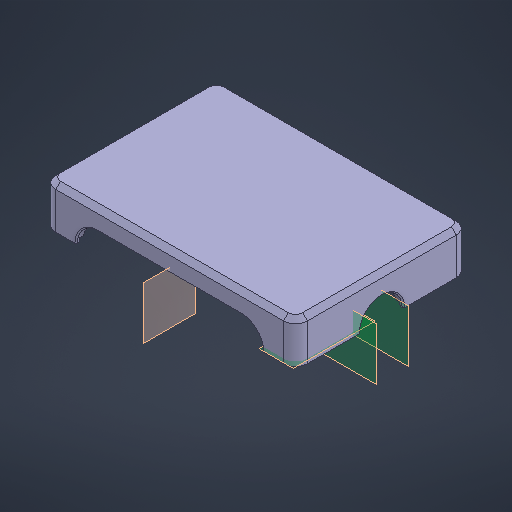
# Autodesk Inventor part: case2
Saved by Autodesk Inventor 2025.2 (Build 292293000, 293)
## iProperties
Created: 2025-10-05
Part Number: case2
Material: Generic
Document SubType Name: Modeling
Designer: micyg
Density: 1 g/cm^3
Appearance: Default
Sheet Metal Rule: Default
Author: micyg
## iProperties of the stored document case2_3DPrint.ipt
Created: 2025-10-05
Part Number: case2_3DPrint
Material: Generic
Document SubType Name: Modeling
Designer: micyg
Density: 1 g/cm^3
Appearance: Default
Author: micyg
Autodesk Inventor part; units mm, degrees
ref_plane "YZ Plane" through (0, 0, 0) normal (1, 0, 0) x (0, 1, 0)
ref_plane "XZ Plane" through (0, 0, 0) normal (0, 1, 0) x (-1, 0, 0)
ref_plane "XY Plane" through (0, 0, 0) normal (0, 0, 1) x (1, 0, 0)
sketch "Sketch1" plane through (0, 0, 0) normal (0, 1, 0) x (-1, 0, 0)
  line L0 (0, 0) -> (105.2, 0)
  line L1 (105.2, 0) -> (105.2, -72.2)
  line L2 (105.2, -72.2) -> (0, -72.2)
  line L3 (0, -72.2) -> (0, 0)
  dimension "d0" = 105.2
  dimension "d1" = 72.2
  constraints: 8 end point, 2 parallel, 1 horizontal, 1 perpendicular
  measures "d0" distance of L1.end L2.end
  measures "d1" distance of L0.end L1.end
extrude "Extrusion1" add sketch "Sketch1" along normal blind 17.5
fillet "Fillet1" radius 5 4 edges at (-105.2, 8.75, 0) (0, 8.75, 0) (-105.2, 8.75, -72.2) (0, 8.75, -72.2)
chamfer "Chamfer1" distance 2 angle 45 8 edges at (-52.6, 17.5, 0) (-1.4645, 17.5, -1.4645) (0, 17.5, -36.1) (-1.4645, 17.5, -70.7355) (-52.6, 17.5, -72.2) (-103.7355, 17.5, -70.7355) (-105.2, 17.5, -36.1) (-103.7355, 17.5, -1.4645)
shell "Shell2" thickness 3 removed faces 1 at (-36.7333, 0, -24.0667)
ref_plane "Work Plane2" through (-52.6, 0, 0) normal (1, 0, 0) x (0, 1, 0)
ref_plane "Work Plane3" through (0, 0, -36.1) normal (0, 0, -1) x (-1, 0, 0)
ref_plane "Work Plane4" through (0, 1.915, 0) normal (0, -1, 0) x (1, 0, 0)
sketch "Sketch19" plane through (-52.6, 0, 0) normal (1, 0, 0) x (0, 1, 0)
  line L0 (0, -3) -> (14.2574, -3) projected
  line L1 (14.2574, -3) -> (0, -3) projected
  line L2 (14.5, -5.7) -> (7.5, -5.7)
  line L3 (6.5, -5.7) -> (7.5, -6.7) construction
  line L4 (7.5, -6.7) -> (7.5, -5.7)
  line L5 (7.5, -5.7) -> (6.5, -5.7) construction
  line L6 (7.5, -6.7) -> (14.5, -13.7)
  line L7 (0, -67.2) -> (0, -72.2) projected
  line L8 (0, -5) -> (0, -67.2) projected
  line L9 (0, 0) -> (0, -5) projected
  line L10 (0, -5) -> (0, 0) projected
  line L11 (0, -67.2) -> (0, -5) projected
  line L12 (0, -72.2) -> (0, -67.2) projected
  line L13 (14.5, -3.2426) -> (14.5, -5) projected
  line L14 (14.5, -5) -> (14.5, -67.2) projected
  line L15 (14.5, -67.2) -> (14.5, -68.9574) projected
  line L16 (14.5, -68.9574) -> (14.5, -67.2) projected
  line L17 (14.5, -67.2) -> (14.5, -5) projected
  line L18 (14.5, -5) -> (14.5, -3.2426) projected
  dimension "d104" = 2.7
  dimension "d105" = 1
  dimension "d157" = 45
  dimension "d179" = 7
  constraints: 10 end point, 2 perpendicular, 2 point on line, 1 collinear
  measures "d104" distance between parallel lines of L0 L2
  measures "d105" distance from line of L3.end L2
  measures "d157" angle of L17 L6
  measures "d179" distance between parallel lines of L17 L4
extrude "Extrusion15" add sketch "Sketch19" against normal up to surface (49.6 mm away)
mirror "Mirror9" about plane through (-52.6, 0, 0) normal (1, 0, 0) of "Extrusion15"
mirror "Mirror10" about plane through (0, 0, -36.1) normal (0, 0, -1) of "Extrusion15", "Mirror9"
sketch "Sketch9" plane through (0, 1.915, 0) normal (0, -1, 0) x (1, 0, 0)
  arc A0 (-5, -72.2) -> (0, -67.2) centre (-5, -67.2) ccw projected
  line L0 (0, -5) -> (0, -67.2) projected
  arc A1 (0, -5) -> (-5, 0) centre (-5, -5) ccw projected
  line L1 (-100.2, 0) -> (-5, 0) projected
  arc A2 (-100.2, 0) -> (-105.2, -5) centre (-100.2, -5) ccw projected
  line L2 (-105.2, -67.2) -> (-105.2, -5) projected
  arc A3 (-105.2, -67.2) -> (-100.2, -72.2) centre (-100.2, -67.2) ccw projected
  line L3 (-5, -72.2) -> (-100.2, -72.2) projected
  line L4 (-5, -70.8) -> (-100.2, -70.8) projected
  arc A4 (-5, -70.8) -> (-1.4, -67.2) centre (-5, -67.2) ccw projected
  line L5 (-1.4, -5) -> (-1.4, -67.2) projected
  arc A5 (-1.4, -5) -> (-5, -1.4) centre (-5, -5) ccw projected
  line L6 (-100.2, -1.4) -> (-5, -1.4) projected
  arc A6 (-100.2, -1.4) -> (-103.8, -5) centre (-100.2, -5) ccw projected
  line L7 (-103.8, -67.2) -> (-103.8, -5) projected
  arc A7 (-103.8, -67.2) -> (-100.2, -70.8) centre (-100.2, -67.2) ccw projected
  line L8 (-102.2, -5) -> (-102.2, -67.2) projected
  arc A8 (-100.2, -3) -> (-102.2, -5) centre (-100.2, -5) ccw projected
  line L9 (-5, -3) -> (-100.2, -3) projected
  arc A9 (-3, -5) -> (-5, -3) centre (-5, -5) ccw projected
  line L10 (-3, -67.2) -> (-3, -5) projected
  arc A10 (-5, -69.2) -> (-3, -67.2) centre (-5, -67.2) ccw projected
  line L11 (-100.2, -69.2) -> (-5, -69.2) projected
  arc A11 (-102.2, -67.2) -> (-100.2, -69.2) centre (-100.2, -67.2) ccw projected
  line L12 (-96.7, -8.6) -> (-8.7, -8.6) construction
  line L13 (-8.7, -8.6) -> (-8.7, -63.6) construction
  line L14 (-8.7, -63.6) -> (-96.7, -63.6) construction
  line L15 (-96.7, -63.6) -> (-96.7, -8.6) construction
  circle A12 centre (-96.7, -8.6) radius 1.5
  circle A13 centre (-8.7, -8.6) radius 1.5
  circle A14 centre (-96.7, -63.6) radius 1.5
  circle A15 centre (-8.7, -63.6) radius 1.5
  line L16 (-52.7, -8.6) -> (-52.7, -63.6) construction
  line L17 (-101.7, -3.6) -> (-3.7, -3.6) construction
  line L18 (-3.7, -3.6) -> (-3.7, -68.6) construction
  line L19 (-3.7, -68.6) -> (-101.7, -68.6) construction
  line L20 (-101.7, -68.6) -> (-101.7, -3.6) construction
  line L21 (-101.7, -36.1) -> (-3.7, -36.1) construction
  line L22 (-52.6, 0) -> (-52.6, -72.2) construction
  line L23 (-105.2, -36.1) -> (0, -36.1) construction
  line L24 (-93.2, -3) -> (-93.2, -8.6)
  line L25 (-102.2, -12.1) -> (-102.2, -5)
  arc A16 (-96.7, -12.1) -> (-93.2, -8.6) centre (-96.7, -8.6) ccw
  line L26 (-96.7, -12.1) -> (-102.2, -12.1)
  line L27 (-100.2, -3) -> (-93.2, -3)
  line L28 (-93.2, -69.2) -> (-93.2, -63.6)
  arc A17 (-93.2, -63.6) -> (-96.7, -60.1) centre (-96.7, -63.6) ccw
  line L29 (-96.7, -60.1) -> (-102.2, -60.1)
  arc A18 (-12.2, -8.6) -> (-8.7, -12.1) centre (-8.7, -8.6) ccw
  line L30 (-3, -12.1) -> (-3, -5)
  line L31 (-12.2, -3) -> (-12.2, -8.6)
  line L32 (-8.7, -12.1) -> (-3, -12.1)
  line L33 (-5, -3) -> (-12.2, -3)
  arc A19 (-8.7, -60.1) -> (-12.2, -63.6) centre (-8.7, -63.6) ccw
  line L34 (-12.2, -69.2) -> (-12.2, -63.6)
  line L35 (-8.7, -60.1) -> (-3, -60.1)
  line L36 (-93.2, -3) -> (-95.2, -3)
  line L37 (-95.2, -3) -> (-95.2, -6)
  line L38 (-95.2, -6) -> (-93.2, -6)
  line L39 (-93.2, -6) -> (-93.2, -3)
  line L40 (-12.2, -3) -> (-10.2, -3)
  line L41 (-10.2, -3) -> (-10.2, -6)
  line L42 (-10.2, -6) -> (-12.2, -6)
  line L43 (-12.2, -6) -> (-12.2, -3)
  line L44 (-95.2, -69.2) -> (-95.2, -66.2)
  line L45 (-95.2, -66.2) -> (-93.2, -66.2)
  line L46 (-10.2, -69.2) -> (-10.2, -66.2)
  line L47 (-10.2, -66.2) -> (-12.2, -66.2)
  arc A20 (-3, -5) -> (-5, -3) centre (-5, -5) ccw projected
  line L48 (-5, -3) -> (-100.2, -3) projected
  arc A21 (-100.2, -3) -> (-102.2, -5) centre (-100.2, -5) ccw projected
  line L49 (-102.2, -5) -> (-102.2, -67.2) projected
  arc A22 (-102.2, -67.2) -> (-100.2, -69.2) centre (-100.2, -67.2) ccw projected
  line L50 (-100.2, -69.2) -> (-5, -69.2) projected
  arc A23 (-5, -69.2) -> (-3, -67.2) centre (-5, -67.2) ccw projected
  line L51 (-3, -67.2) -> (-3, -5) projected
  arc A24 (0, -5) -> (-5, 0) centre (-5, -5) ccw projected
  line L52 (0, -5) -> (0, -67.2) projected
  arc A25 (-5, -72.2) -> (0, -67.2) centre (-5, -67.2) ccw projected
  line L53 (-5, -72.2) -> (-100.2, -72.2) projected
  arc A26 (-105.2, -67.2) -> (-100.2, -72.2) centre (-100.2, -67.2) ccw projected
  line L54 (-105.2, -67.2) -> (-105.2, -5) projected
  arc A27 (-100.2, 0) -> (-105.2, -5) centre (-100.2, -5) ccw projected
  line L55 (-100.2, 0) -> (-5, 0) projected
  arc A28 (-3, -5) -> (-5, -3) centre (-5, -5) ccw projected
  line L56 (-5, -3) -> (-100.2, -3) projected
  arc A29 (-100.2, -3) -> (-102.2, -5) centre (-100.2, -5) ccw projected
  line L57 (-102.2, -5) -> (-102.2, -67.2) projected
  arc A30 (-102.2, -67.2) -> (-100.2, -69.2) centre (-100.2, -67.2) ccw projected
  line L58 (-100.2, -69.2) -> (-5, -69.2) projected
  arc A31 (-5, -69.2) -> (-3, -67.2) centre (-5, -67.2) ccw projected
  line L59 (-3, -67.2) -> (-3, -5) projected
  arc A32 (0, -5) -> (-5, 0) centre (-5, -5) ccw projected
  line L60 (0, -5) -> (0, -67.2) projected
  arc A33 (-5, -72.2) -> (0, -67.2) centre (-5, -67.2) ccw projected
  line L61 (-5, -72.2) -> (-100.2, -72.2) projected
  arc A34 (-105.2, -67.2) -> (-100.2, -72.2) centre (-100.2, -67.2) ccw projected
  line L62 (-105.2, -67.2) -> (-105.2, -5) projected
  arc A35 (-100.2, 0) -> (-105.2, -5) centre (-100.2, -5) ccw projected
  line L63 (-100.2, 0) -> (-5, 0) projected
  point P0 (-52.7, -36.1)
  dimension "d137" = 88
  dimension "d138" = 55
  dimension "d139" = 3
  dimension "d140" = 3
  dimension "d141" = 3
  dimension "d142" = 3
  dimension "d143" = 98
  dimension "d144" = 65
  dimension "d145" = 0.5
  dimension "d147" = 2
  dimension "d148" = 2
  dimension "d149" = 3
  dimension "d150" = 2
  constraints: 72 end point, 16 symmetric about line, 12 parallel, 12 point on circle, 10 midpoint, 8 centre point, 6 horizontal, 6 perpendicular, 6 point on line, 5 coincident, 4 tangent, 1 collinear, 3 other
  measures "d137" distance of L12.start L12.end
  measures "d138" distance of L14.end L12.start
  measures "d139" diameter of A12
  measures "d140" diameter of A15
  measures "d141" diameter of A13
  measures "d142" diameter of A14
  measures "d143" distance of L17.start L17.end
  measures "d144" distance of L19.end L17.start
  measures "d145" distance between parallel lines of L8 L20
  measures "d147" radial gap between concentric circles of A12 A16
  measures "d148" radial gap between concentric circles of A18 A13
  measures "d149" distance between parallel lines of L9 L38
  measures "d150" distance between parallel lines of L24 L37
extrude "Extrusion13" add sketch "Sketch9" against normal up to surface (12.585 mm away) contours A8 L9 L37 L38 L24 A16 L26 L8 | L29 A17 L28 L45 L44 L11 A11 L8 | L9 A9 L10 L32 A18 L31 L42 L41 | L46 L47 L34 A19 L35 L10 A10 L11 | A12 | A13 | A14 | A15
ref_plane "Work Plane6" through (0, 0, -24.1) normal (0, 0, -1) x (-1, 0, 0)
sketch "Sketch22" plane through (0, 0, -24.1) normal (0, 0, -1) x (-1, 0, 0)
  line L0 (3, 2.5) -> (15, 14.5)
  line L1 (90.2, 14.5) -> (102.2, 2.5)
  line L2 (3, 1.915) -> (3, 12.9) projected
  line L3 (3, 12.9) -> (3, 1.915) projected
  line L4 (3, 1.915) -> (3, 0) projected
  line L5 (3, 0) -> (3, 1.915) projected
  line L6 (3.2426, 14.5) -> (101.9574, 14.5) projected
  line L7 (101.9574, 14.5) -> (3.2426, 14.5) projected
  line L8 (102.2, 14.2574) -> (101.9574, 14.5) projected
  line L9 (101.9574, 14.5) -> (102.2, 14.2574) projected
  line L10 (102.2, 1.915) -> (102.2, 12.9) projected
  line L11 (102.2, 12.9) -> (102.2, 1.915) projected
  line L12 (102.2, 1.915) -> (102.2, 0) projected
  line L13 (102.2, 0) -> (102.2, 1.915) projected
  line L14 (52.6, -3.5) -> (52.6, 21) projected
  line L15 (102.2, 12.9) -> (102.2, 14.2574) projected
  line L16 (102.2, 14.2574) -> (102.2, 12.9) projected
  line L17 (3.2426, 14.5) -> (3, 14.2574) projected
  line L18 (3, 14.2574) -> (3.2426, 14.5) projected
  line L19 (3, 12.9) -> (3, 14.2574) projected
  line L20 (3, 14.2574) -> (3, 12.9) projected
  point P0 (102.2, 14.2574)
  dimension "d184" = 12
  dimension "d185" = 45
  constraints: 4 end point, 4 point on line, 1 other
  measures "d184" distance from line of L6 L0.start
  measures "d185" angle of L7 L0
extrude "Extrusion18" add sketch "Sketch22" along normal mid plane 2
mirror "Mirror12" about plane through (0, 0, -36.1) normal (0, 0, -1) of "Extrusion18"
sketch "Sketch26" plane through (0, 1.915, 0) normal (0, -1, 0) x (1, 0, 0)
  line L0 (-95.2, -69.2) -> (-10.2, -69.2) projected
  line L1 (-5, -69.2) -> (-10.2, -69.2) projected
  arc A0 (-5, -69.2) -> (-3, -67.2) centre (-5, -67.2) ccw projected
  line L2 (-3, -67.2) -> (-3, -60.1) projected
  line L3 (-3, -60.1) -> (-3, -12.1) projected
  line L4 (0, -5) -> (0, -67.2) projected
  arc A1 (-5, -72.2) -> (0, -67.2) centre (-5, -67.2) ccw projected
  line L5 (-5, -72.2) -> (-100.2, -72.2) projected
  line L6 (-10.2, -69.2) -> (-10.2, -66.2) projected
  line L7 (-10.2, -66.2) -> (-12.2, -66.2) projected
  line L8 (-12.2, -66.2) -> (-12.2, -63.6) projected
  arc A2 (-8.7, -60.1) -> (-12.2, -63.6) centre (-8.7, -63.6) ccw projected
  line L9 (-8.7, -60.1) -> (-3, -60.1) projected
  line L10 (-10.2, -6) -> (-10.2, -3) projected
  line L11 (-10.2, -3) -> (-5, -3) projected
  arc A3 (-3, -5) -> (-5, -3) centre (-5, -5) ccw projected
  line L12 (-3, -12.1) -> (-3, -5) projected
  arc A4 (0, -5) -> (-5, 0) centre (-5, -5) ccw projected
  line L13 (-100.2, 0) -> (-5, 0) projected
  line L14 (-10.2, -3) -> (-95.2, -3) projected
  line L15 (-12.2, -6) -> (-10.2, -6) projected
  line L16 (-12.2, -8.6) -> (-12.2, -6) projected
  arc A5 (-12.2, -8.6) -> (-8.7, -12.1) centre (-8.7, -8.6) ccw projected
  line L17 (-3, -12.1) -> (-8.7, -12.1) projected
  line L18 (-95.2, -3) -> (-95.2, -6) projected
  line L19 (-95.2, -6) -> (-93.2, -6) projected
  line L20 (-93.2, -6) -> (-93.2, -8.6) projected
  arc A6 (-96.7, -12.1) -> (-93.2, -8.6) centre (-96.7, -8.6) ccw projected
  line L21 (-96.7, -12.1) -> (-102.2, -12.1) projected
  line L22 (-102.2, -5) -> (-102.2, -12.1) projected
  arc A7 (-100.2, -3) -> (-102.2, -5) centre (-100.2, -5) ccw projected
  line L23 (-100.2, -3) -> (-95.2, -3) projected
  arc A8 (-100.2, 0) -> (-105.2, -5) centre (-100.2, -5) ccw projected
  line L24 (-105.2, -67.2) -> (-105.2, -5) projected
  arc A9 (-105.2, -67.2) -> (-100.2, -72.2) centre (-100.2, -67.2) ccw projected
  line L25 (-95.2, -69.2) -> (-100.2, -69.2) projected
  arc A10 (-102.2, -67.2) -> (-100.2, -69.2) centre (-100.2, -67.2) ccw projected
  line L26 (-102.2, -60.1) -> (-102.2, -67.2) projected
  line L27 (-102.2, -12.1) -> (-102.2, -60.1) projected
  line L28 (-95.2, -66.2) -> (-95.2, -69.2) projected
  line L29 (-93.2, -66.2) -> (-95.2, -66.2) projected
  line L30 (-93.2, -63.6) -> (-93.2, -66.2) projected
  arc A11 (-93.2, -63.6) -> (-96.7, -60.1) centre (-96.7, -63.6) ccw projected
  line L31 (-102.2, -60.1) -> (-96.7, -60.1) projected
  circle A12 centre (-96.7, -63.6) radius 1.5 projected
  circle A13 centre (-96.7, -8.6) radius 1.5 projected
  circle A14 centre (-8.7, -8.6) radius 1.5 projected
  circle A15 centre (-8.7, -63.6) radius 1.5 projected
  point P0 (0, 0)
extrude "Extrusion21" cut sketch "Sketch26" against normal up to surface (12.585 mm away) contours A12 | A13 | A14 | A15
sketch "Sketch30" plane through (0, 0, -5) normal (1, 0, 0) x (0, 0, -1)
  line L0 (0, 15.5) -> (62.2, 15.5) construction
  line L1 (0, 0) -> (0, 15.5) construction
  line L2 (0, 0) -> (62.2, 0) construction
  line L3 (62.2, 15.5) -> (62.2, 0) construction
  line L4 (31.1, 22.8) -> (31.1, -14.3) construction
  circle A0 centre (31.1, 0) radius 9
  point P0 (-5, 0)
  dimension "d160" = 18
  constraints: 1 centre point, 1 midpoint, 1 point on line
  measures "d160" diameter of A0
extrude "Extrusion22" cut sketch "Sketch30" against normal up to surface (3 mm away)
sketch "Sketch31" plane through (-5, 0, -72.2) normal (0, 0, -1) x (-1, 0, 0)
  line L0 (17.7, -9) -> (47.6, -9)
  arc A0 (17.7, 9) -> (17.7, -9) centre (17.7, 0) ccw
  line L1 (54.189, 9) -> (17.7, 9)
  line L2 (77.7, -9) -> (47.6, -9)
  arc A1 (77.7, -9) -> (77.7, 9) centre (77.7, 0) ccw
  line L3 (54.189, 9) -> (77.7, 9)
  line L4 (86.7, 9) -> (8.7, 9) construction
  line L5 (8.7, 9) -> (8.7, -9) construction
  line L6 (8.7, -9) -> (86.7, -9) construction
  line L7 (86.7, -9) -> (86.7, 9) construction
  line L8 (86.7, 9) -> (8.7, -9) construction
  line L9 (8.7, 9) -> (86.7, -9) construction
  line L10 (0, 15.5) -> (95.2, 15.5) projected
  line L11 (0, 0) -> (0, 15.5) projected
  line L12 (0, 0) -> (95.2, 0) projected
  line L13 (95.2, 15.5) -> (95.2, 0) projected
  line L14 (47.6, -14.3) -> (47.6, 22.8) projected
  point P0 (47.7, 0)
  point P1 (47.7, 0)
  point P2 (47.7, 0)
  dimension "d163" = 9
  dimension "d164" = 78
  dimension "d168" = 0.1
  constraints: 20 end point, 6 tangent, 4 midpoint, 4 point on circle, 3 collinear, 3 parallel, 3 point on line, 2 centre point, 1 horizontal, 1 perpendicular
  measures "d163" radius of A0
  measures "d164" distance between parallel lines of L5 L7
  measures "d168" distance from line of L14 point (47.7, 0)
extrude "Extrusion23" cut sketch "Sketch31" against normal up to surface (3 mm away) contours A0 L12 L14 L0 | L14 L12 A1 L2 | A0 L1 L14 L12 | L14 L1 L3 A1 L12
mirror "Mirror13" about plane through (0, 0, -36.1) normal (0, 0, -1) of "Extrusion23"
sketch "Sketch33" plane through (0, 0, 0) normal (0, -1, 0) x (1, 0, 0)
  line L0 (-91.7, -3) -> (-91.7, 0) projected
  line L1 (-100.2, 0) -> (-91.7, 0) projected
  arc A0 (-100.2, 0) -> (-105.2, -5) centre (-100.2, -5) ccw projected
  line L2 (-105.2, -67.2) -> (-105.2, -5) projected
  arc A1 (-105.2, -67.2) -> (-100.2, -72.2) centre (-100.2, -67.2) ccw projected
  line L3 (-91.7, -72.2) -> (-100.2, -72.2) projected
  line L4 (-91.7, -72.2) -> (-91.7, -69.2) projected
  line L5 (-91.7, -69.2) -> (-100.2, -69.2) projected
  arc A2 (-102.2, -67.2) -> (-100.2, -69.2) centre (-100.2, -67.2) ccw projected
  line L6 (-102.2, -67.2) -> (-102.2, -5) projected
  arc A3 (-100.2, -3) -> (-102.2, -5) centre (-100.2, -5) ccw projected
  line L7 (-100.2, -3) -> (-91.7, -3) projected
  line L8 (-13.7, 0) -> (-13.7, -3) projected
  line L9 (-13.7, -3) -> (-5, -3) projected
  arc A4 (-3, -5) -> (-5, -3) centre (-5, -5) ccw projected
  line L10 (-3, -5) -> (-3, -27.1) projected
  line L11 (-3, -27.1) -> (0, -27.1) projected
  line L12 (0, -5) -> (0, -27.1) projected
  arc A5 (0, -5) -> (-5, 0) centre (-5, -5) ccw projected
  line L13 (-13.7, 0) -> (-5, 0) projected
  line L14 (-13.7, -69.2) -> (-13.7, -72.2) projected
  line L15 (-5, -72.2) -> (-13.7, -72.2) projected
  arc A6 (-5, -72.2) -> (0, -67.2) centre (-5, -67.2) ccw projected
  line L16 (0, -45.1) -> (0, -67.2) projected
  line L17 (0, -45.1) -> (-3, -45.1) projected
  line L18 (-3, -45.1) -> (-3, -67.2) projected
  arc A7 (-5, -69.2) -> (-3, -67.2) centre (-5, -67.2) ccw projected
  line L19 (-5, -69.2) -> (-13.7, -69.2) projected
  arc A8 (-5, -70.8) -> (-1.4, -67.2) centre (-5, -67.2) ccw
  line L20 (-5, -70.8) -> (-13.7, -70.8)
  line L21 (-1.4, -45.1) -> (-1.4, -67.2)
  line L22 (-13.7, -1.4) -> (-5, -1.4)
  arc A9 (-1.4, -5) -> (-5, -1.4) centre (-5, -5) ccw
  line L23 (-1.4, -5) -> (-1.4, -27.1)
  line L24 (-103.8, -5) -> (-103.8, -67.2)
  arc A10 (-103.8, -67.2) -> (-100.2, -70.8) centre (-100.2, -67.2) ccw
  line L25 (-100.2, -70.8) -> (-91.7, -70.8)
  line L26 (-91.7, -1.4) -> (-100.2, -1.4)
  arc A11 (-100.2, -1.4) -> (-103.8, -5) centre (-100.2, -5) ccw
  line L27 (-13.7, 0) -> (-13.7, -3) projected
  line L28 (-91.7, -72.2) -> (-91.7, -69.2) projected
  line L29 (-91.7, -3) -> (-91.7, 0) projected
  line L30 (-3, -45.1) -> (-3, -27.1) projected
  line L31 (-1.4, -45.1) -> (-3, -45.1)
  line L32 (-3, -45.1) -> (-3, -27.1)
  line L33 (-3, -27.1) -> (-1.4, -27.1)
  line L34 (-1.4, -27.1) -> (-1.4, -45.1)
  line L35 (-91.7, -1.4) -> (-13.7, -1.4)
  line L36 (-13.7, -1.4) -> (-13.7, -3)
  line L37 (-13.7, -3) -> (-91.7, -3)
  line L38 (-91.7, -3) -> (-91.7, -1.4)
  line L39 (-5, -69.2) -> (-13.7, -69.2) projected
  line L40 (-13.7, -69.2) -> (-91.7, -69.2)
  line L41 (-91.7, -69.2) -> (-91.7, -70.8)
  line L42 (-91.7, -70.8) -> (-13.7, -70.8)
  line L43 (-13.7, -70.8) -> (-13.7, -69.2)
  point P0 (0, 0)
  dimension "d174" = 1.4
  dimension "d175" = 1.4
  dimension "d176" = 1.4
  constraints: 38 end point, 8 point on circle, 6 parallel, 6 point on line, 4 centre point, 3 horizontal, 3 perpendicular, 2 tangent, 6 other
  measures "d174" distance between parallel lines of L1 L26
  measures "d175" distance between parallel lines of L13 L22
  measures "d176" distance between parallel lines of L16 L21
extrude "Extrusion25" cut sketch "Sketch33" against normal blind 1.6 contours L7 A3 L6 A2 L5 L4 L25 A10 L24 A11 L26 L0 | L0 L35 L8 L37 | L8 L22 A9 L23 L11 L10 A4 L9 | L11 L34 L17 L30 | L40 L14 L42 L4 | L17 L21 A8 L20 L14 L19 A7 L18
sketch "Sketch34" plane through (0, 0, -25.1) normal (0, 0, -1) x (-1, 0, 0)
  line L0 (3, 14.2574) -> (3, 2.5) projected
  line L1 (3.2426, 14.5) -> (3, 14.2574) projected
  line L2 (15, 14.5) -> (3.2426, 14.5) projected
  line L3 (15, 14.5) -> (3, 2.5) construction
  line L4 (101.9574, 14.5) -> (90.2, 14.5) projected
  line L5 (90.2, 14.5) -> (101.9574, 14.5) projected
  line L6 (101.9574, 14.5) -> (3.2426, 14.5) projected
  line L7 (3.2426, 14.5) -> (15, 14.5) projected
  line L8 (15, 14.5) -> (3.2426, 14.5) projected
  line L9 (3.2426, 14.5) -> (15, 14.5) projected
  line L10 (15, 14.5) -> (3.2426, 14.5) projected
  line L11 (3.2426, 14.5) -> (101.9574, 14.5) projected
  line L12 (101.9574, 14.5) -> (90.2, 14.5) projected
  line L13 (90.2, 14.5) -> (101.9574, 14.5) projected
  line L14 (5.6, 14.5) -> (5.6, 7.5)
  line L15 (5.6, 6.5) -> (6.6, 7.5) construction
  line L16 (5.6, 7.5) -> (6.6, 7.5)
  line L17 (6.6, 7.5) -> (13.6, 14.5)
  line L18 (5.6, 7.5) -> (5.6, 6.5) construction
  point P0 (0, 0)
  dimension "d180" = 1
  dimension "d181" = 45
  dimension "d182" = 7
  dimension "d183" = 2.6
  constraints: 10 end point, 2 point on line, 2 vertical, 1 collinear, 1 horizontal
  measures "d180" distance from line of L15.end L14
  measures "d181" angle of L11 L17
  measures "d182" distance between parallel lines of L6 L16
  measures "d183" distance between parallel lines of L0 L14
extrude "Extrusion26" add sketch "Sketch34" along normal up to surface (22 mm away)
chamfer "Chamfer2" distance 0.5 angle 45 7 edges at (-16.336, 6.364, 0) (-52.7, 9, 0) (-89.064, 6.364, 0) (-16.336, 6.364, -72.2) (-52.7, 9, -72.2) (-89.064, 6.364, -72.2) (0, 9, -36.1)
equation "\"BendRadius\" = Thickness"
equation "\"BendReliefWidth\" = Thickness"
equation "\"BendReliefDepth\" = 0.5 * Thickness"
equation "\"CornerReliefSize\" = 4 * Thickness"
equation "\"MinimumRemnant\" = 2 * Thickness"
equation "\"TransitionRadius\" = BendRadius"
equation "\"JacobiRadiusSize\" = BendRadius"
equation "\"GapSize\" = Thickness"
equation "\"Thickness\" = 3.048"
body "Solid1"
